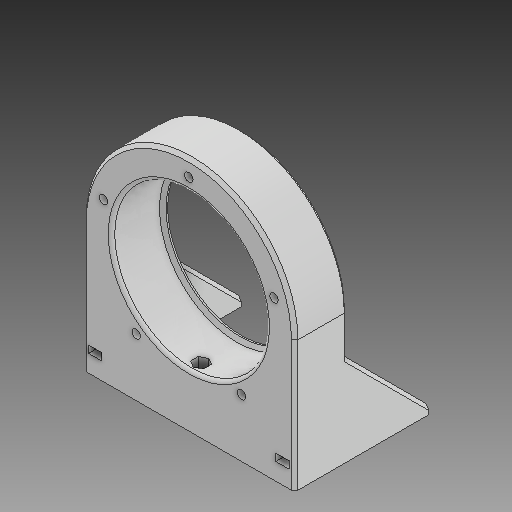
# Autodesk Inventor part: J1_idlebracket
Saved by Autodesk Inventor 2020 (Build 240168000, 168)
## iProperties
Created: 2021-03-20
Part Number: J1_idlebracket
Material: Generic
Document SubType Name: Modeling
Designer: DDeGo
Density: 1 g/cm^3
Appearance: Default
Author: DDeGo
Autodesk Inventor part; units mm, degrees
ref_plane "YZ Plane" through (0, 0, 0) normal (1, 0, 0) x (0, 1, 0)
ref_plane "XZ Plane" through (0, 0, 0) normal (0, 1, 0) x (-1, 0, 0)
ref_plane "XY Plane" through (0, 0, 0) normal (0, 0, 1) x (1, 0, 0)
sketch "Sketch1" plane through (0, 0, 0) normal (0, 0, 1) x (1, 0, 0)
  circle A0 centre (0, 0) radius 47.525
  arc A1 (65, 0) -> (-65, 0) centre (0, 0) ccw
  line L0 (-65, 0) -> (-65, -80)
  line L1 (-65, -80) -> (65, -80)
  line L2 (65, -80) -> (65, 0)
  dimension "d0" = 95.05
  dimension "d2" = 80
  dimension "d43" = 65
  constraints: 6 end point, 2 centre point, 2 coincident, 2 point on circle, 2 tangent, 2 vertical, 1 perpendicular
  measures "d0" diameter of A0
  measures "d2" distance from line of L1 point (0, 0)
  measures "d43" radius of A1
extrude "Extrusion1" add sketch "Sketch1" along normal blind 32.5
sketch "Sketch2" plane through (0, 0, 0) normal (0, 0, -1) x (-1, 0, 0)
  circle A0 centre (0, 0) radius 47.525 projected
  circle A1 centre (0, 0) radius 45.525
  dimension "d5" = 2
  constraints: 1 centre point, 1 coincident
  measures "d5" radial gap between concentric circles of A0 A1
extrude "Extrusion2" add sketch "Sketch2" against normal blind 1
sketch "Sketch3" plane through (0, 0, 32.5) normal (0, 0, 1) x (1, 0, 0)
  arc A0 (65, 0) -> (-65, 0) centre (0, 0) ccw construction
  line L0 (0, 0) -> (0, 55) construction
  circle A1 centre (0, 55) radius 2.6
  circle A2 centre (-52.3081, 16.9959) radius 2.6
  circle A3 centre (-32.3282, -44.4959) radius 2.6
  circle A4 centre (32.3282, -44.4959) radius 2.6
  circle A5 centre (52.3081, 16.9959) radius 2.6
  dimension "d8" = 5.2
  dimension "d9" = 55
  dimension "d12" = 360
  constraints: 5 centre point, 5 coincident, 2 end point, 1 vertical, 16 other
  measures "d8" diameter of A1
  measures "d9" distance of L0.start L0.end
extrude "Extrusion3" cut sketch "Sketch3" against normal through all
sketch "Sketch7" plane through (-65, -80, 0) normal (-1, 0, 0) x (0, 0, 1)
  line L0 (0, 0) -> (32.5, 0) projected
  line L1 (0, 0) -> (-50, 0)
  line L2 (-50, 0) -> (-50, 5)
  line L3 (0, 80) -> (0, 0) projected
  line L4 (-50, 5) -> (0, 55)
  line L5 (0, 0) -> (0, 55)
  dimension "d32" = 50
  dimension "d33" = 5
  dimension "d34" = 135
  constraints: 8 end point, 2 parallel, 1 horizontal, 1 point on line
  measures "d32" distance of L0.start L1.end
  measures "d33" distance of L1.end L2.end
  measures "d34" angle of L2 L4
extrude "Extrusion7" add sketch "Sketch7" against normal blind 15
mirror "Mirror1" about plane through (0, 0, 0) normal (1, 0, 0) of "Extrusion7"
sketch "Sketch5" plane through (-65, -80, 0) normal (0, -1, 0) x (1, 0, 0)
  circle A0 centre (7.5, 25) radius 2.75
  circle A1 centre (122.5, 25) radius 2.75
  circle A2 centre (93.75, 7.5) radius 2.75
  circle A3 centre (36.25, 7.5) radius 2.75
  circle A4 centre (65, 25) radius 2.75
  line L0 (7.5, 25) -> (65, 25) construction
  line L1 (65, 25) -> (122.5, 25) construction
  line L2 (93.75, 7.5) -> (36.25, 7.5) construction
  line L3 (65, 25) -> (65, 7.5) construction
  line L4 (65, 7.5) -> (65, 0) construction
  line L5 (0, 0) -> (130, 0) construction
  line L6 (0, 32.5) -> (130, 32.5) construction
  line L7 (0, 0) -> (0, 32.5) construction
  line L8 (36.25, 25) -> (36.25, 7.5) construction
  line L9 (0, -50) -> (15, -50) construction
  line L10 (7.5, -50) -> (7.5, -40) construction
  line L11 (130, -50) -> (115, -50) construction
  line L12 (122.5, -50) -> (122.5, -40) construction
  line L13 (122.5, -40) -> (7.5, -40) construction
  circle A5 centre (7.5, -40) radius 2.75
  circle A6 centre (122.5, -40) radius 2.75
  line L14 (122.5, -40) -> (122.5, 25) construction
  line L15 (130, -50) -> (130, 32.5) projected
  dimension "d16" = 5.5
  dimension "d17" = 7.5
  dimension "d18" = 7.5
  dimension "d37" = 10
  dimension "d39" = 17.5
  dimension "d45" = 57.5
  dimension "d46" = 65
  dimension "d47" = 7.5
  constraints: 20 end point, 7 centre point, 6 equal radius, 6 vertical, 4 midpoint, 3 horizontal, 2 coincident, 1 collinear, 1 perpendicular
  measures "d16" diameter of A0
  measures "d17" distance between parallel lines of L5 L2
  measures "d18" distance between parallel lines of L6 L0
  measures "d37" distance of L10.start L10.end
  measures "d39" distance of L8.start L2.end
  measures "d45" distance of L0.end L1.end
  measures "d46" distance of L14.start L1.end
  measures "d47" distance between parallel lines of L15 L14
extrude "Extrusion4" cut sketch "Sketch5" against normal blind 18
ref_plane "Work Plane1" through (-65, -65, 0) normal (0, -1, 0) x (1, 0, 0)
sketch "Sketch6" plane through (-65, -65, 0) normal (0, -1, 0) x (1, 0, 0)
  circle A0 centre (122.5, 25) radius 2.75 projected
  circle A1 centre (65, 25) radius 2.75 projected
  circle A2 centre (36.25, 7.5) radius 2.75 projected
  line L0 (122.5, 29.7343) -> (126.6, 27.3671) construction
  line L1 (126.6, 27.3671) -> (126.6, 22.6329)
  line L2 (126.6, 22.6329) -> (122.5, 20.2657)
  line L3 (122.5, 20.2657) -> (118.4, 22.6329)
  line L4 (118.4, 22.6329) -> (118.4, 27.3671)
  line L5 (118.4, 27.3671) -> (122.5, 29.7343) construction
  line L6 (65, 29.7343) -> (69.1, 27.3671)
  line L7 (69.1, 27.3671) -> (69.1, 22.6329)
  line L8 (69.1, 22.6329) -> (65, 20.2657)
  line L9 (65, 20.2657) -> (60.9, 22.6329)
  line L10 (60.9, 22.6329) -> (60.9, 27.3671)
  line L11 (60.9, 27.3671) -> (65, 29.7343)
  circle A3 centre (36.25, 7.5) radius 2.75 projected
  line L12 (36.25, 2.7657) -> (32.15, 5.1329) construction
  line L13 (32.15, 5.1329) -> (32.15, 9.8671)
  line L14 (32.15, 9.8671) -> (36.25, 12.2343)
  line L15 (36.25, 12.2343) -> (40.35, 9.8671)
  line L16 (40.35, 9.8671) -> (40.35, 5.1329)
  line L17 (40.35, 5.1329) -> (36.25, 2.7657) construction
  circle A4 centre (93.75, 7.5) radius 2.75 projected
  line L18 (93.75, 2.7657) -> (89.65, 5.1329) construction
  line L19 (89.65, 5.1329) -> (89.65, 9.8671)
  line L20 (89.65, 9.8671) -> (93.75, 12.2343)
  line L21 (93.75, 12.2343) -> (97.85, 9.8671)
  line L22 (97.85, 9.8671) -> (97.85, 5.1329)
  line L23 (97.85, 5.1329) -> (93.75, 2.7657) construction
  circle A5 centre (7.5, 25) radius 2.75 projected
  line L24 (7.5, 20.2657) -> (3.4, 22.6329)
  line L25 (3.4, 22.6329) -> (3.4, 27.3671)
  line L26 (3.4, 27.3671) -> (7.5, 29.7343) construction
  line L27 (7.5, 29.7343) -> (11.6, 27.3671) construction
  line L28 (11.6, 27.3671) -> (11.6, 22.6329)
  line L29 (11.6, 22.6329) -> (7.5, 20.2657)
  line L30 (126.6, 27.3671) -> (126.6, 35.5137)
  line L31 (126.6, 35.5137) -> (118.4, 35.5137)
  line L32 (118.4, 35.5137) -> (118.4, 27.3671)
  line L33 (97.85, 5.1329) -> (97.85, -3.3085)
  line L34 (97.85, -3.3085) -> (89.65, -3.3085)
  line L35 (89.65, -3.3085) -> (89.65, 5.1329)
  line L36 (40.35, 5.1329) -> (40.35, -3.965)
  line L37 (40.35, -3.965) -> (32.15, -3.965)
  line L38 (32.15, -3.965) -> (32.15, 5.1329)
  line L39 (17.475, 1) -> (112.525, 1) projected
  line L40 (11.6, 27.3671) -> (11.6, 33.5607)
  line L41 (11.6, 33.5607) -> (3.4, 33.5607)
  line L42 (3.4, 33.5607) -> (3.4, 27.3671)
  circle A6 centre (122.5, -40) radius 2.75 projected
  circle A7 centre (122.5, -40) radius 2.75 projected
  circle A8 centre (7.5, -40) radius 2.75 projected
  line L43 (122.5, -44.7343) -> (118.4, -42.3671)
  line L44 (118.4, -42.3671) -> (118.4, -37.6329)
  line L45 (118.4, -37.6329) -> (122.5, -35.2657)
  line L46 (122.5, -35.2657) -> (126.6, -37.6329)
  line L47 (126.6, -37.6329) -> (126.6, -42.3671)
  line L48 (126.6, -42.3671) -> (122.5, -44.7343)
  line L49 (7.5, -44.7343) -> (3.4, -42.3671)
  line L50 (3.4, -42.3671) -> (3.4, -37.6329)
  line L51 (3.4, -37.6329) -> (7.5, -35.2657)
  line L52 (7.5, -35.2657) -> (11.6, -37.6329)
  line L53 (11.6, -37.6329) -> (11.6, -42.3671)
  line L54 (11.6, -42.3671) -> (7.5, -44.7343)
  point P0 (65, 0)
  point P1 (40.35, 1)
  point P2 (32.15, 1)
  point P3 (97.85, 1)
  point P4 (89.65, 1)
  dimension "d23" = 8.2
  constraints: 108 end point, 11 vertical, 7 coincident, 6 equal length, 5 perpendicular, 3 collinear, 91 other
  measures "d23" distance between parallel lines of L4 L1
extrude "Extrusion5" cut sketch "Sketch6" along normal blind 4.5 contours A1 | L1 L2 L3 L4 L32 L31 L30 | L6 L7 L8 L9 L10 L11 | L13 L14 L15 L16 L36 L39 L38 | L39 L36 L37 L38 | L19 L20 L21 L22 L33 L39 L35 | L39 L33 L34 L35 | L24 L25 L42 L41 L40 L28 L29 | L43 L44 L45 L46 L47 L48 | L49 L50 L51 L52 L53 L54
extrude "Extrusion6" cut sketch "Sketch6" against normal blind 20.75 contours A1 | L6 L7 L8 L9 L10 L11 | L43 L44 L45 L46 L47 L48 | L49 L50 L51 L52 L53 L54
fillet "Fillet1" radius 2 1 edges at (-47.525, 0, 32.5)
chamfer "Chamfer1" distance 2 angle 45 10 edges at (0, 65, 32.5) (-65, -40, 32.5) (65, -40, 32.5) (0, 65, 0) (-65, -12.5, 0) (65, -12.5, 0) (-65, -50, -25) (-50, -50, -25) (50, -50, -25) (65, -50, -25)
fillet "Fillet2" radius 5 4 edges at (-50, -53.9142, 0) (50, -53.9142, 0) (57.5, -25, 0) (-57.5, -25, 0)
chamfer "Chamfer2" distance 2 angle 45 1 edges at (-47.525, 0, 1)
equation "\"d17\" = d47"
equation "\"d18\" = d47"
body "Solid1"
